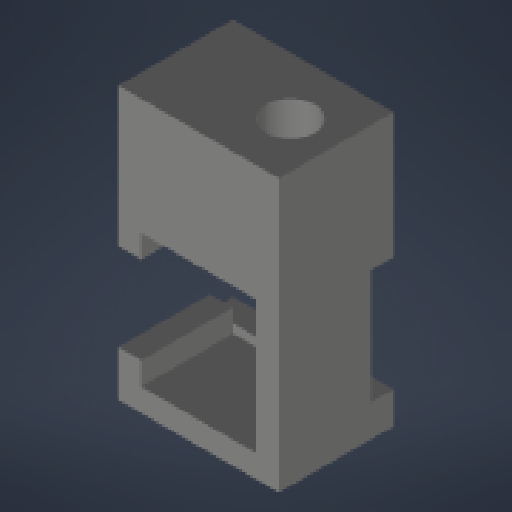
# Autodesk Inventor part: Adafruit_1528_4663-ND_House_02
Saved by Autodesk Inventor 2026.2 (Build 302298000, 298)
## iProperties
Created: 2026-02-03
Part Number: Adafruit_1528_4663-ND_House_02
Material: Generic
Document SubType Name: Modeling
Designer: vckot
Density: 1 g/cm^3
Appearance: Gray
Author: vckot
Autodesk Inventor part; units mm, degrees
ref_plane "YZ Plane" through (0, 0, 0) normal (1, 0, 0) x (0, 1, 0)
ref_plane "XZ Plane" through (0, 0, 0) normal (0, 1, 0) x (-1, 0, 0)
ref_plane "XY Plane" through (0, 0, 0) normal (0, 0, 1) x (1, 0, 0)
sketch "Sketch1" plane through (0, 0, 0) normal (0, 0, 1) x (1, 0, 0)
  line L0 (-6.25, -7.25) -> (6.25, -7.25)
  line L1 (6.25, -7.25) -> (6.25, 7.25)
  line L2 (6.25, 7.25) -> (-6.25, 7.25)
  line L3 (-6.25, 7.25) -> (-6.25, -7.25)
  line L4 (-6.25, -7.25) -> (6.25, 7.25) construction
  line L5 (6.25, -7.25) -> (-6.25, 7.25) construction
  line L6 (-8.75, -9.75) -> (8.75, -9.75)
  line L7 (8.75, -9.75) -> (8.75, 9.75)
  line L8 (8.75, 9.75) -> (-8.75, 9.75)
  line L9 (-8.75, 9.75) -> (-8.75, -9.75)
  line L10 (-8.75, -9.75) -> (8.75, 9.75) construction
  line L11 (8.75, -9.75) -> (-8.75, 9.75) construction
  point P0 (0, 0)
  dimension "d0" = 12.5
  dimension "d1" = 14.5
  dimension "d2" = 17.5
  dimension "d3" = 19.5
  constraints: 24 end point, 4 midpoint, 4 parallel, 2 horizontal, 2 perpendicular
  measures "d0" distance of L2.end L1.end
  measures "d1" distance of L1.end L0.end
  measures "d2" distance of L7.end L8.end
  measures "d3" distance of L6.end L7.end
extrude "Extrusion1" add sketch "Sketch1" along normal blind 10
sketch "Sketch2" plane through (0, 0, 0) normal (0, 0, -1) x (-1, 0, 0)
  line L0 (8.75, 9.75) -> (8.75, -9.75) projected
  line L1 (-8.75, 9.75) -> (8.75, 9.75)
  line L2 (8.75, 9.75) -> (8.75, 6.25)
  line L3 (8.75, 6.25) -> (-8.75, 6.25)
  line L4 (-8.75, 6.25) -> (-8.75, 9.75)
  line L5 (6.25, 7.25) -> (-6.25, 7.25) projected
  line L6 (-8.75, -9.75) -> (-8.75, 9.75) projected
  line L7 (-8.75, -9.75) -> (8.75, -9.75)
  line L8 (8.75, -9.75) -> (8.75, -6.25)
  line L9 (8.75, -6.25) -> (-8.75, -6.25)
  line L10 (-8.75, -6.25) -> (-8.75, -9.75)
  line L11 (-6.25, -7.25) -> (6.25, -7.25) projected
  point P0 (0, 0)
  point P1 (-8.75, -6.25)
  dimension "d6" = 1
  dimension "d7" = 1
  constraints: 16 end point, 4 parallel, 2 horizontal, 2 perpendicular, 2 point on line
  measures "d6" distance between parallel lines of L5 L3
  measures "d7" distance between parallel lines of L9 L11
extrude "Extrusion2" add sketch "Sketch2" along normal blind 2.5 contours L0 L3 L4 L1 | L0 L7 L6 L9
thicken "Thicken1" operation add thickness 10.199 both sides no extend neighbours no toward (0, 1, 0) faces at (-2.9167, 9.75, 5.8333)
sketch "Sketch3" plane through (-8.75, 19.949, 10) normal (0, 1, 0) x (1, 0, 0)
  line L0 (0, 12.5) -> (0, 0) projected
  line L1 (17.5, 12.5) -> (17.5, 0) projected
  point P0 (8.75, 10)
  point P1 (12.5, 6.25)
  point P2 (0, 6.25)
  dimension "d19" = 5
  constraints: 1 horizontal alignment, 1 midpoint
  measures "d19" distance from line of L1 point (12.5, 6.25)
hole "Hole1" at (3.75, 19.949, 3.75) direction (0, -1, 0) diameter 5.35 depth 10 tip angle 118
sketch "Sketch4" plane through (-8.75, -6.25, 0) normal (-1, 0, 0) x (0, 0, 1)
  line L0 (10, -3.5) -> (10, 26.199) projected
  line L1 (0, 12.5) -> (0, 0) projected
  line L2 (10, 1.5) -> (0, 1.5)
  line L3 (0, 1.5) -> (0, 11)
  line L4 (0, 11) -> (10, 11)
  line L5 (10, 11) -> (10, 1.5)
  line L6 (-2.5, -3.5) -> (10, -3.5) projected
  point P0 (0, 6.25)
  point P1 (0, 1.5)
  dimension "d20" = 5
  dimension "d21" = 9.5
  constraints: 8 end point, 2 parallel, 2 point on line, 1 horizontal, 1 perpendicular
  measures "d20" distance between parallel lines of L6 L2
  measures "d21" distance between parallel lines of L4 L2
extrude "Extrusion3" cut sketch "Sketch4" against normal blind 5
body "Solid1"
